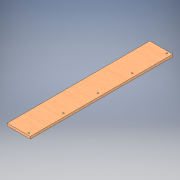
# Autodesk Inventor part: support-pinces
Saved by Autodesk Inventor 2019 (Build 230136000, 136)
## iProperties
Created: 2020-02-15
Part Number: support-pinces
Material: Generic
Document SubType Name: Modeling
Designer: franc
Density: 1 g/cm^3
Appearance: Default
Author: franc
Autodesk Inventor part; units mm, degrees
ref_plane "YZ Plane" through (0, 0, 0) normal (1, 0, 0) x (0, 1, 0)
ref_plane "XZ Plane" through (0, 0, 0) normal (0, 1, 0) x (-1, 0, 0)
ref_plane "XY Plane" through (0, 0, 0) normal (0, 0, 1) x (1, 0, 0)
sketch "Esquisse1" plane through (0, 0, 0) normal (0, 1, 0) x (-1, 0, 0)
  line L0 (48.408, 155.3632) -> (-1.592, 155.3632)
  line L1 (-1.592, 155.3632) -> (-1.592, -154.6368)
  line L2 (-1.592, -154.6368) -> (48.408, -154.6368)
  line L3 (48.408, -154.6368) -> (48.408, 155.3632)
  point P0 (0, 0)
  dimension "d0" = 310
  dimension "d1" = 50
  constraints: 8 end point, 2 parallel, 1 horizontal, 1 perpendicular
  measures "d0" distance of L2.end L0.start
  measures "d1" distance of L1.end L2.end
extrude "Extrusion1" add sketch "Esquisse1" along normal blind 5
sketch "Esquisse2" plane through (0, 5, 0) normal (0, 1, 0) x (1, 0, 0)
  circle A0 centre (-6.408, -75.3632) radius 1.5
  circle A1 centre (-6.408, -0.3632) radius 1.5
  circle A2 centre (-6.408, 74.6368) radius 1.5
  line L0 (1.592, -155.3632) -> (1.592, 154.6368) projected
  line L1 (-48.408, -155.3632) -> (1.592, -155.3632) projected
  circle A3 centre (-6.408, -150.3632) radius 1.5
  circle A4 centre (-6.408, 149.6368) radius 1.5
  point P0 (0, 0)
  dimension "d5" = 3
  dimension "d6" = 3
  dimension "d8" = 3
  dimension "d10" = 8
  dimension "d11" = 8
  dimension "d13" = 8
  dimension "d14" = 155
  dimension "d15" = 75
  dimension "d16" = 75
  dimension "d17" = 3
  dimension "d18" = 8
  dimension "d19" = 75
  dimension "d20" = 3
  dimension "d21" = 8
  dimension "d22" = 75
  constraints: 5 centre point
  measures "d5" diameter of A0
  measures "d6" diameter of A1
  measures "d8" diameter of A2
  measures "d10" distance from line of L0 A0.centre
  measures "d11" distance from line of L0 A1.centre
  measures "d13" distance from line of L0 A2.centre
  measures "d14" distance from line of L1 A1.centre
  measures "d15" distance of A0.centre A1.centre
  measures "d16" distance of A2.centre A1.centre
  measures "d17" diameter of A3
  measures "d18" distance from line of L0 A3.centre
  measures "d19" distance of A3.centre A0.centre
  measures "d20" diameter of A4
  measures "d21" distance from line of L0 A4.centre
  measures "d22" distance of A4.centre A2.centre
extrude "Extrusion2" cut sketch "Esquisse2" against normal through all
